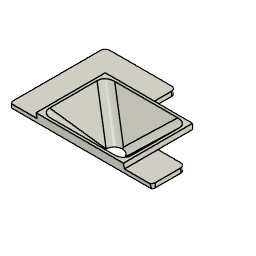
smartie_hopper (Autodesk Fusion 360 design; units mm, degrees)
part number: 2025-05-19-10-29-37-314
Autodesk Fusion 360 part; units mm, degrees
sketch "Bottom opening" plane through (0, 0, 0) normal (0, 0, 1) x (1, 0, 0)
  line L0 (0, 0) -> (18, 0)
  line L1 (18, 0) -> (18, 18)
  line L2 (18, 18) -> (0, 18)
  line L3 (0, 18) -> (0, 0)
  line L4 (-4, 22) -> (22, 22)
  line L5 (22, 22) -> (22, -4)
  line L6 (22, -4) -> (-4, -4)
  line L7 (-4, -4) -> (-4, 22)
  dimension "d3" = 18
  dimension "d4" = 18
  dimension "d5" = 4
  dimension "d6" = 4
  dimension "d7" = 4
  dimension "d8" = 4
  constraint horizontal L0
  constraint vertical L1
  constraint horizontal L2
  constraint vertical L3
  constraint coincident L0.start L3.end
  constraint horizontal L4
  constraint vertical L5
  constraint horizontal L6
  constraint vertical L7
  measures "d3" distance of L0.start L0.end
  measures "d4" distance of L0.end L1.end
  measures "d5" distance of L2 L4
  measures "d6" distance of L0 L6
  measures "d7" distance of L1 L5
  measures "d8" distance of L3 L7
ref_plane "WorkPlane1" through (0, 0, 34) normal (0, 0, 1) x (1, 0, 0)
sketch "Top opening" plane through (0, 0, 34) normal (0, 0, 1) x (1, 0, 0)
  line L0 (18, 18) -> (0, 18)
  line L1 (18, 0) -> (18, 18)
  line L2 (0, 0) -> (18, 0)
  line L3 (0, 18) -> (0, 0)
  line L4 (-4, 22) -> (22, 22)
  line L5 (22, -4) -> (-4, -4)
  line L6 (22, 22) -> (22, -4)
  line L7 (-4, -4) -> (-4, 22)
  line L8 (-36, 44) -> (54, 44)
  line L9 (54, 44) -> (54, -26)
  line L10 (54, -26) -> (-36, -26)
  line L11 (-36, -26) -> (-36, 44)
  line L12 (-39, 47) -> (57, 47)
  line L13 (57, 47) -> (57, -29)
  line L14 (57, -29) -> (-39, -29)
  line L15 (-39, -29) -> (-39, 47)
  line L16 (-40, 48) -> (58, 48)
  line L17 (58, 48) -> (58, -30)
  line L18 (58, -30) -> (-40, -30)
  line L19 (-40, -30) -> (-40, 48)
  dimension "d14" = 3
  dimension "d15" = 4
  dimension "d16" = 3
  dimension "d17" = 4
  dimension "d18" = 90
  dimension "d19" = 70
  dimension "d20" = 3
  dimension "d21" = 4
  dimension "d22" = 3
  dimension "d23" = 4
  dimension "d24" = 32
  dimension "d25" = 32
  dimension "d26" = 22
  dimension "d27" = 22
  constraint horizontal L8
  constraint vertical L9
  constraint horizontal L10
  constraint vertical L11
  constraint horizontal L12
  constraint vertical L13
  constraint horizontal L14
  constraint vertical L15
  constraint horizontal L16
  constraint vertical L17
  constraint horizontal L18
  constraint vertical L19
  measures "d14" distance of L9 L13
  measures "d15" distance of L9 L17
  measures "d16" distance of L11 L15
  measures "d17" distance of L11 L19
  measures "d18" distance of L8.start L8.end
  measures "d19" distance of L8.end L9.end
  measures "d20" distance of L8 L12
  measures "d21" distance of L8 L16
  measures "d22" distance of L10 L14
  measures "d23" distance of L10 L18
  measures "d24" distance of L7 L11
  measures "d25" distance of L6 L9
  measures "d26" distance of L4 L8
  measures "d27" distance of L5 L10
loft "Loft1" add profiles "Top opening", "Bottom opening" section 1 contours L8 L9 L10 L11 | L12 L13 L14 L15 | L16 L17 L18 L19 section 2 contours L0 L1 L2 L3 | L4 L5 L6 L7
extrude "Extrude1" cut sketch "Top opening" against normal blind 6 contours L16 L17 L18 L19
extrude "Extrude4" add 1 faces at (25, -3.6667, 34) along direction (0, 0, -1) blind 6
sketch "Support lip" plane through (57, 0, 0) normal (1, 0, 0) x (0, 1, 0)
  line L0 (47, 28) -> (47, 34)
  line L1 (47, 34) -> (-29, 34)
  line L2 (-29, 34) -> (-29, 28)
  line L3 (-29, 28) -> (77, 28)
  line L4 (77, 28) -> (77, 23)
  line L5 (77, 23) -> (-29, 23)
  line L6 (-29, 23) -> (-29, 28)
  line L7 (-29, 28) -> (47, 28)
  line L8 (-29, 28) -> (9, 28)
  line L9 (9, 28) -> (9, 23)
  line L10 (9, 23) -> (-29, 23)
  line L11 (-29, 23) -> (-29, 28)
  dimension "d31" = 6
  dimension "d34" = 5
  dimension "d35" = 30
  dimension "d50" = 38
  constraint horizontal L3
  constraint vertical L4
  constraint horizontal L5
  constraint vertical L6
  constraint collinear L2 L6
  constraint horizontal L8
  constraint vertical L9
  constraint horizontal L10
  constraint vertical L11
  constraint coincident L5 L9.end
  constraint coincident L2.end L3.start
  measures "d31" distance of L1 L3
  measures "d34" distance of L2.end L5.end
  measures "d35" horizontal distance of L0.end L3.end
  measures "d50" distance of L9 L11
extrude "Extrude2" add sketch "Support lip" along normal blind 30 and the other way blind 126 contours L3 L5 L6 L7 L8 L9 L10 L11
extrude "Extrude5" add sketch "Support lip" against normal blind 78 from surface at -48 contours L3 L4 L5 L7 L9
fillet "Fillet4" radius 5 5 edges at (87, 9, 25.5) (87, -29, 25.5) (9, 77, 25.5) (-69, 77, 25.5) (-69, -29, 25.5)
loft "Loft2" cut profiles "Top opening", "Bottom opening" section 1 contours L8 L9 L10 L11 section 2 contours L0 L1 L2 L3
fillet "Fillet3" radius 12.803 4 edges at (-18, 31, 17) (-18, -13, 17) (36, -13, 17) (36, 31, 17)
fillet "Fillet5" radius 18.495 4 edges at (-16.1765, -12.7941, 11.5) (-16.1765, 30.7941, 11.5) (36.8235, 32.7059, 14) (34.1765, -12.7941, 11.5)
sketch "3D printing angle" plane through (87, 0, 0) normal (1, 0, 0) x (0, 1, 0)
  line L0 (-24, 28) -> (-24, 23)
  line L1 (-24, 23) -> (4, 23)
  line L2 (4, 23) -> (4, 28)
  line L3 (4, 28) -> (-24, 28)
  line L4 (47, 28) -> (47, 34)
  line L5 (47, 34) -> (-29, 34)
  line L6 (-29, 34) -> (-29, 28)
  line L7 (-29, 28) -> (9, 28)
  line L8 (9, 28) -> (47, 28)
  line L9 (-24, 23) -> (-29, 23)
  line L10 (-24, 23) -> (-24, 28)
  line L11 (-29, 28) -> (-24, 28)
  line L12 (-29, 28) -> (-29, 23)
  line L13 (4, 28) -> (9, 28)
  line L14 (4, 28) -> (4, 23)
  line L15 (9, 23) -> (4, 23)
  line L16 (9, 23) -> (9, 28)
  line L17 (-29, 34) -> (-27.0604, 23)
  dimension "d58" = 10
  constraint coincident L5.end L6.start
  constraint coincident L9 L17.end
  measures "d58" angle of L6 L17
extrude "Extrude6" cut sketch "3D printing angle" against normal blind 156 contours L7 L9 L11 L12 L17 | L6 L7 L11 L17
equation "bottom_outlet_size = 18 mm" comment "The side lengths of the bottom opening of the Smartie Hopper."
equation "hopper_wall_thickness = 4 mm" comment "The thickness of the hopper walls used for the \"loft\" function."
equation "d3 = bottom_outlet_size"
equation "d4 = bottom_outlet_size"
equation "d5 = hopper_wall_thickness"
equation "d6 = hopper_wall_thickness"
equation "d7 = hopper_wall_thickness"
equation "d8 = hopper_wall_thickness"
equation "hopper_height = 34 mm" comment "Distance between the top and bottom openings of the Smartie Hopper."
equation "d10 = hopper_height"
equation "acrylic_thickness = 3 mm" comment "Thickness of the clear acrylic panels used for the Unsorted Smarties Holder."
equation "top_outlet_width = 90 mm" comment "The width of the top opening of the Smartie Hopper."
equation "top_outlet_depth = 70 mm" comment "The depth of the top opening of the Smartie Hopper."
equation "d14 = acrylic_thickness"
equation "d15 = hopper_wall_thickness"
equation "d16 = acrylic_thickness"
equation "d17 = hopper_wall_thickness"
equation "d18 = top_outlet_width"
equation "d19 = top_outlet_depth"
equation "d20 = acrylic_thickness"
equation "d21 = hopper_wall_thickness"
equation "d22 = acrylic_thickness"
equation "d23 = hopper_wall_thickness"
equation "d24 = ( top_outlet_width - ( bottom_outlet_size + 2 * hopper_wall_thickness ) ) / 2"
equation "d26 = ( top_outlet_depth - ( bottom_outlet_size + 2 * hopper_wall_thickness ) ) / 2"
equation "MDF_thickness = 6 mm" comment "Thickness of the MDF panels used for the construction of the mini arcade game enclosure."
equation "d29 = -MDF_thickness"
equation "d31 = MDF_thickness"
equation "support_lip_width = 30 mm" comment "The depth that the suport lip should extend beneath the Colour Detection Mechanism Top Panel."
equation "support_lip_thickness = 5 mm" comment "The thickness of the support lip."
equation "d34 = support_lip_thickness"
equation "d35 = support_lip_width"
equation "d36 = support_lip_width"
equation "d38 = ( top_outlet_width + 2 * acrylic_thickness ) + support_lip_width"
equation "d46 = -MDF_thickness"
equation "d50 = ( top_outlet_depth / 2 ) + acrylic_thickness"
equation "d51 = -( top_outlet_width / 2 ) - acrylic_thickness"
equation "d52 = -( top_outlet_width / 2 ) - acrylic_thickness - support_lip_width"
equation "d59 = -( top_outlet_width + 2 * acrylic_thickness + 2 * support_lip_width )"
named bodies: "Smartie Hopper"
